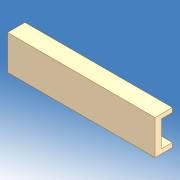
# Autodesk Inventor part: NASA-20-EBOX-SEXTC-01
Saved by Autodesk Inventor 2020 (Build 240168000, 168)
## iProperties
Created: 2019-10-09
Part Number: NASA-20-EBOX-SEXTC-01
Material: Polyethylene, Low Density
Document SubType Name: Modeling
Designer: mpark
Density: 0.894 g/cm^3
Appearance: White
Author: mpark
Autodesk Inventor part; units mm, degrees
ref_plane "YZ Plane" through (0, 0, 0) normal (1, 0, 0) x (0, 1, 0)
ref_plane "XZ Plane" through (0, 0, 0) normal (0, 1, 0) x (-1, 0, 0)
ref_plane "XY Plane" through (0, 0, 0) normal (0, 0, 1) x (1, 0, 0)
sketch "Sketch1" plane through (0, 0, 0) normal (1, 0, 0) x (0, 1, 0)
  line L0 (0, 0) -> (50.8, 0)
  line L1 (50.8, 0) -> (50.8, -25.4)
  line L2 (50.8, -25.4) -> (44.45, -25.4)
  line L3 (44.45, -25.4) -> (44.45, -9.525)
  line L4 (44.45, -9.525) -> (6.35, -9.525)
  line L5 (6.35, -9.525) -> (6.35, -25.4)
  line L6 (6.35, -25.4) -> (0, -25.4)
  line L7 (0, -25.4) -> (0, 0)
  dimension "d1" = 15.875
  dimension "d3" = 6.35
  dimension "d4" = 6.35
  dimension "d5" = 50.8
  dimension "d9" = 25.4
  constraints: 16 end point, 6 perpendicular, 2 point on line, 1 horizontal
  measures "d1" distance of L4.end L5.end
  measures "d3" distance of L5.end L6.end
  measures "d4" distance of L1.end L2.end
  measures "d5" distance of L0.start L0.end
  measures "d9" distance between parallel lines of L6 L0
extrude "Extrusion1" add sketch "Sketch1" along normal blind 215.9
body "Solid1"
